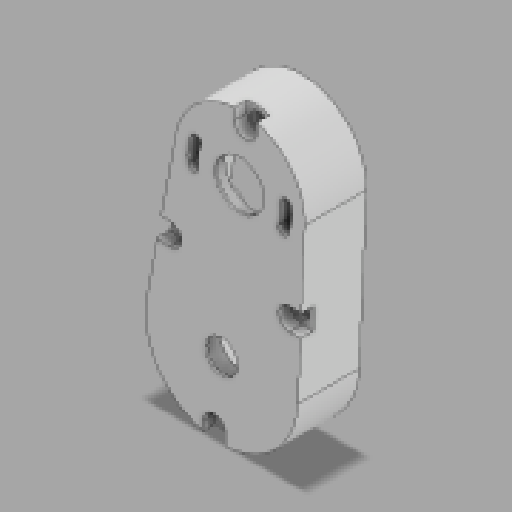
# Autodesk Inventor part: Верх редуктора
Saved by Autodesk Inventor 2025 (Build 290162000, 162)
## iProperties
Created: 2025-04-09
Part Number: Верх редуктора
Material: Типовые
Document SubType Name: Modeling
Designer: Artem Sannikov
Density: 1 g/cm^3
Appearance: По умолчанию
Author: Artem Sannikov
Autodesk Inventor part; units mm, degrees
ref_plane "YZ Plane" through (0, 0, 0) normal (1, 0, 0) x (0, 1, 0)
ref_plane "XZ Plane" through (0, 0, 0) normal (0, 1, 0) x (-1, 0, 0)
ref_plane "XY Plane" through (0, 0, 0) normal (0, 0, 1) x (1, 0, 0)
sketch "Эскиз1" plane through (0, 0, 0) normal (0, 0, 1) x (1, 0, 0)
  arc A0 (-29.2789, -52.5351) -> (18.293, -57.9783) centre (-5.684, -56.9258) ccw projected
  line L0 (18.293, -57.9783) -> (20.4803, -8.149) projected
  arc A1 (20.4803, -8.149) -> (-20.154, -3.4996) centre (0, -7.25) ccw projected
  line L1 (-20.154, -3.4996) -> (-29.2789, -52.5351) projected
  circle A2 centre (0, -7.25) radius 9.5 projected
  circle A3 centre (-5.684, -56.9258) radius 7.5 projected
  point P0 (0, 0)
extrude "Выдавливание1" add sketch "Эскиз1" against normal blind 4
sketch "Эскиз2" plane through (0, 0, -4) normal (0, 0, -1) x (-1, 0, 0)
  circle A0 centre (5.684, -56.9258) radius 7.5 projected
  circle A1 centre (5.684, -56.9258) radius 10
  point P0 (0, 0)
  dimension "d2" = 20
  constraints: 1 centre point, 1 coincident
  measures "d2" diameter of A1
extrude "Выдавливание2" add sketch "Эскиз2" along normal blind 2
sketch "Эскиз3" plane through (0, 0, 0) normal (0, 0, 1) x (1, 0, 0)
  line L0 (18.293, -57.9783) -> (20.4803, -8.149) projected
  arc A0 (20.4803, -8.149) -> (-20.154, -3.4996) centre (0, -7.25) ccw projected
  line L1 (-20.154, -3.4996) -> (-29.2789, -52.5351) projected
  arc A1 (-29.2789, -52.5351) -> (18.293, -57.9783) centre (-5.684, -56.9258) ccw projected
  circle A2 centre (-5.684, -56.9258) radius 5.1702
  circle A3 centre (0, -7.25) radius 7.692
  point P0 (0, 0)
  constraints: 2 centre point, 2 coincident
extrude "Выдавливание3" add sketch "Эскиз3" along normal blind 0.7
sketch "Эскиз4" plane through (0, 0, -4) normal (0, 0, -1) x (-1, 0, 0)
  line L0 (-20.4803, -8.149) -> (-19.6493, -27.0798) projected
  line L1 (-18.293, -57.9783) -> (-19.6493, -27.0798) projected
  arc A0 (-18.293, -57.9783) -> (29.2789, -52.5351) centre (5.684, -56.9258) ccw projected
  line L2 (23.6207, -22.1288) -> (29.2789, -52.5351) projected
  line L3 (20.154, -3.4996) -> (23.6207, -22.1288) projected
  arc A1 (20.154, -3.4996) -> (-20.4803, -8.149) centre (0, -7.25) ccw projected
  line L4 (-17.6512, -26.9921) -> (-18.4822, -8.0613)
  arc A2 (18.1878, -3.8655) -> (-18.4822, -8.0613) centre (0, -7.25) ccw
  line L5 (18.1878, -3.8655) -> (21.6544, -22.4947)
  line L6 (21.6544, -22.4947) -> (27.3127, -52.901)
  arc A3 (-16.2949, -57.8906) -> (27.3127, -52.901) centre (5.684, -56.9258) ccw
  line L7 (-16.2949, -57.8906) -> (-17.6512, -26.9921)
  point P0 (0, 0)
  dimension "d7" = 2
  constraints: 8 end point, 4 point on circle, 2 centre point, 5 other
  measures "d7" distance between parallel lines of L0 L4
ref_plane "РабПлоскость1" through (-56.4021, -90.7621, -18.8) normal (0, 0, 1) x (0.81648, -0.5773737, 0)
extrude "Выдавливание4" add sketch "Эскиз4" along normal up to surface (14.8 mm away)
sketch "Эскиз5" plane through (0, 0, 0.7) normal (0, 0, 1) x (1, 0, 0)
  arc A0 (12.2361, -11.9701) -> (12.9958, -5.4859) centre (0, -7.25) ccw projected
  arc A1 (12.2361, -11.9701) -> (15.315, -13.1578) centre (13.7756, -12.564) ccw projected
  arc A2 (16.2658, -5.042) -> (12.9958, -5.4859) centre (14.6308, -5.2639) ccw projected
  arc A3 (15.315, -13.1578) -> (16.2658, -5.042) centre (0, -7.25) ccw projected
  arc A4 (-12.2362, -2.5298) -> (-12.9958, -9.0141) centre (0, -7.25) ccw projected
  arc A5 (-12.2362, -2.5298) -> (-15.315, -1.3422) centre (-13.7756, -1.936) ccw projected
  arc A6 (-16.2658, -9.458) -> (-12.9958, -9.0141) centre (-14.6308, -9.2361) ccw projected
  arc A7 (-15.315, -1.3422) -> (-16.2658, -9.458) centre (0, -7.25) ccw projected
  point P0 (0, 0)
extrude "Выдавливание5" cut sketch "Эскиз5" against normal blind 8
sketch "Эскиз6" plane through (0, 0, 0.7) normal (0, 0, 1) x (1, 0, 0)
  arc A0 (-29.2789, -52.5351) -> (18.293, -57.9783) centre (-5.684, -56.9258) ccw projected
  arc A1 (20.4803, -8.149) -> (-20.154, -3.4996) centre (0, -7.25) ccw projected
  line L0 (-20.154, -3.4996) -> (-29.2789, -52.5351) projected
  line L1 (18.293, -57.9783) -> (20.4803, -8.149) projected
  line L2 (-8.4123, -80.7702) -> (2.3304, 13.1171) construction
  circle A2 centre (-7.986, -77.0445) radius 3.75
  circle A3 centre (1.9041, 9.3914) radius 3.75
  line L3 (-4.236, -77.0445) -> (-4.236, -80.8821)
  line L4 (-11.736, -77.0445) -> (-11.736, -80.1502)
  line L5 (5.6541, 9.3914) -> (5.6541, 12.4548)
  line L6 (-1.8459, 9.3914) -> (-1.8459, 13.1667)
  line L7 (-3.0409, -33.8266) -> (25.9823, -37.1474) construction
  line L8 (-3.0409, -33.8266) -> (-37.3599, -29.8997) construction
  circle A4 centre (-21.5882, -31.7044) radius 3.75
  circle A5 centre (15.5064, -35.9488) radius 3.75
  line L9 (-21.5882, -27.9544) -> (-24.7165, -28.0173)
  line L10 (15.5064, -32.1988) -> (19.417, -32.3704)
  line L11 (15.5064, -39.6988) -> (19.0885, -39.856)
  line L12 (-22.0145, -35.43) -> (-26.0108, -34.9728)
  point P0 (0, 0)
  dimension "d12" = 7.5
  dimension "d13" = 7.5
  dimension "d14" = 7.5
  dimension "d15" = 7.5
  constraints: 22 end point, 14 point on circle, 8 tangent, 7 point on line, 4 centre point, 4 parallel, 3 perpendicular, 2 midpoint, 1 vertical
  measures "d12" diameter of A2
  measures "d13" diameter of A3
  measures "d14" diameter of A4
  measures "d15" diameter of A5
extrude "Выдавливание6" cut sketch "Эскиз6" against normal blind 4 contours L10 L1 A5 | A4 | L4 A2 A0 | L0 A4 L12 | A2 L3 A0 | A2 | L0 L9 A4 | L11 A5 L1 | A1 A3 L6 | A5 | A1 L5 A3 | A3
sketch "Эскиз7" plane through (0, 0, -3.3) normal (0, 0, 1) x (1, 0, 0)
  arc A0 (-22.0145, -35.43) -> (-21.5882, -27.9544) centre (-21.5882, -31.7044) ccw projected
  circle A1 centre (-21.5882, -31.7044) radius 2.25
  arc A2 (-4.236, -77.0445) -> (-11.736, -77.0445) centre (-7.986, -77.0445) ccw projected
  circle A3 centre (-7.986, -77.0445) radius 2.25
  arc A4 (15.5064, -32.1988) -> (15.5064, -39.6988) centre (15.5064, -35.9488) ccw projected
  circle A5 centre (15.5064, -35.9488) radius 2.25
  arc A6 (-1.8459, 9.3914) -> (5.6541, 9.3914) centre (1.9041, 9.3914) ccw projected
  circle A7 centre (1.9041, 9.3914) radius 2.25
  point P0 (0, 0)
  dimension "d18" = 4.5
  dimension "d19" = 4.5
  dimension "d20" = 4.5
  dimension "d21" = 4.5
  constraints: 4 centre point, 4 coincident
  measures "d18" diameter of A1
  measures "d19" diameter of A3
  measures "d20" diameter of A5
  measures "d21" diameter of A7
extrude "Выдавливание7" cut sketch "Эскиз7" against normal through all
sketch "Эскиз8" plane through (0, 0, -4) normal (0, 0, -1) x (-1, 0, 0)
  arc A0 (-17.1927, -37.4383) -> (-17.3167, -34.6126) centre (-15.5064, -35.9488) ccw projected
  arc A1 (-17.3167, -34.6126) -> (-17.1927, -37.4383) centre (-15.5064, -35.9488) ccw projected
  arc A2 (-0.6209, 11.2396) -> (-3.5717, 10.9019) centre (-1.9041, 9.3914) ccw projected
  arc A3 (-3.5717, 10.9019) -> (-0.6209, 11.2396) centre (-1.9041, 9.3914) ccw projected
  arc A4 (23.0499, -29.9938) -> (23.5674, -32.7745) centre (21.5882, -31.7044) ccw projected
  arc A5 (23.5674, -32.7745) -> (23.0499, -29.9938) centre (21.5882, -31.7044) ccw projected
  arc A6 (9.643, -78.5666) -> (6.7156, -78.9016) centre (7.986, -77.0445) ccw projected
  arc A7 (6.7156, -78.9016) -> (9.643, -78.5666) centre (7.986, -77.0445) ccw projected
  arc A8 (-15.5064, -39.6988) -> (-15.5064, -32.1988) centre (-15.5064, -35.9488) ccw projected
  circle A9 centre (-15.5064, -35.9488) radius 3.75
  circle A10 centre (-1.9041, 9.3914) radius 3.5
  circle A11 centre (21.5882, -31.7044) radius 3.5
  circle A12 centre (7.986, -77.0445) radius 3.5
  point P0 (0, 0)
  constraints: 4 coincident, 3 centre point, 3 other
ref_plane "РабПлоскость2" through (-56.4021, -90.7621, -18.8) normal (0, 0, 1) x (0.81648, -0.5773737, 0)
extrude "Выдавливание8" add sketch "Эскиз8" along normal up to surface (14.8 mm away)
